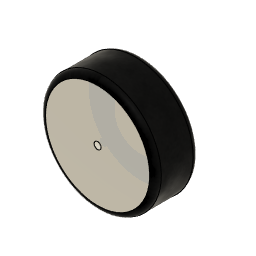
Robot v42 (Autodesk Fusion 360 archive; units mm, degrees)
design "Roues"
Autodesk Fusion 360 part; units mm, degrees
sketch "Esquisse1" plane through (0, 0, 0) normal (0, 1, 0) x (1, 0, 0)
  circle A0 centre (0, 0) radius 20
  circle A1 centre (0, 0) radius 3.1
  line L0 (-2.1, -2.2804) -> (-2.1, 2.2804)
  line L1 (2.1, -2.2804) -> (2.1, 2.2804)
  line L2 (0, 0) -> (0, -3.1) construction
  line L3 (0, 0) -> (0, 3.1) construction
  dimension "d1" = 40
  dimension "d4" = 6.2
  dimension "d5" = 4.2
  constraint coincident A0.centre A1.centre
  constraint concentric A0 A1
  constraint coincident A1 L0.start
  constraint coincident A1 L0.end
  constraint vertical L0
  constraint coincident A1 L1.start
  constraint coincident A1 L1.end
  constraint parallel L0 L1
  constraint coincident A1 L2.end
  constraint parallel L1 L2
  constraint coincident A1 L3.end
  constraint parallel L2 L3
  constraint symmetric L0 L1 L2
  measures "d1" diameter of A0
  measures "d4" diameter of A1
  measures "d5" distance of L0 L1
extrude "Extrusion1" add sketch "Esquisse1" along normal blind 7 contours A0 | A1 L1 | A1 L0
sketch "Esquisse2" plane through (0, 0, 0) normal (0, -1, 0) x (1, 0, 0)
  arc A0 (2.1, 2.2804) -> (-2.1, 2.2804) centre (0, 0) ccw
  line L0 (2.1, 2.2804) -> (2.1, -2.2804)
  arc A1 (-2.1, -2.2804) -> (2.1, -2.2804) centre (0, 0) ccw
  line L1 (-2.1, -2.2804) -> (-2.1, 2.2804)
  circle A2 centre (0, 0) radius 20
  constraint coincident A0.centre A1.centre
extrude "Extrusion2" add sketch "Esquisse2" against normal blind 4 contours A0 L0 A1 L1
hole "Perçage1" at (0, 0, 0) direction (0, 1, 0) diameter 2.4 depth 23 tip angle 118
sketch "Esquisse3" plane through (0, 7, 0) normal (0, 1, 0) x (-1, 0, 0)
  arc A0 (2.1, 2.2804) -> (-2.1, 2.2804) centre (0, 0) ccw
  line L0 (2.1, 2.2804) -> (2.1, -2.2804)
  arc A1 (-2.1, -2.2804) -> (2.1, -2.2804) centre (0, 0) ccw
  line L1 (-2.1, -2.2804) -> (-2.1, 2.2804)
  circle A2 centre (0, 0) radius 20
  arc A3 (2.1, 2.2804) -> (-2.1, 2.2804) centre (0, 0) ccw
  line L2 (-2.1, 2.2804) -> (-2.1, -2.2804)
  arc A4 (-2.1, -2.2804) -> (2.1, -2.2804) centre (0, 0) ccw
  line L3 (2.1, -2.2804) -> (2.1, 2.2804)
  arc A5 (-3.1, -2.6833) -> (3.1, -2.6833) centre (0, 0) ccw
  line L4 (3.1, 2.6833) -> (3.1, -2.6833)
  arc A6 (3.1, 2.6833) -> (-3.1, 2.6833) centre (0, 0) ccw
  line L5 (-3.1, -2.6833) -> (-3.1, 2.6833)
  circle A7 centre (0, 0) radius 1.2
  dimension "d11" = -1
extrude "Extrusion3" add sketch "Esquisse3" along normal blind 6 contours A5 L4 A6 L5
fillet "Congé1" radius 2 4 edges at (3.1, 10, 2.6833) (3.1, 10, -2.6833) (-3.1, 10, 2.6833) (-3.1, 10, -2.6833)
fillet "Congé2" radius 6 8 edges at (3.1, 7, 0) (2.8457, 7, 2.7648) (0, 7, 4.1) (-2.8457, 7, 2.7648) (-3.1, 7, 0) (-2.8457, 7, -2.7648) (0, 7, -4.1) (2.8457, 7, -2.7648)
sketch "Esquisse4" plane through (0, 7, 0) normal (0, 1, 0) x (-1, 0, 0)
  circle A0 centre (0, 0) radius 20
  line L0 (-9.1, -1.7889) -> (-9.1, 1.7889)
  arc A1 (-5.2905, 8.6035) -> (-9.1, 1.7889) centre (-1.1, 1.7889) ccw
  arc A2 (5.2905, 8.6035) -> (-5.2905, 8.6035) centre (0, 0) ccw
  arc A3 (9.1, 1.7889) -> (5.2905, 8.6035) centre (1.1, 1.7889) ccw
  line L1 (9.1, 1.7889) -> (9.1, -1.7889)
  arc A4 (5.2905, -8.6035) -> (9.1, -1.7889) centre (1.1, -1.7889) ccw
  arc A5 (-5.2905, -8.6035) -> (5.2905, -8.6035) centre (0, 0) ccw
  arc A6 (-9.1, -1.7889) -> (-5.2905, -8.6035) centre (-1.1, -1.7889) ccw
  circle A7 centre (0, 0) radius 20
  circle A8 centre (0, 0) radius 10.25
  line L2 (0, 0) -> (0, 20) construction
  line L3 (0, 10.25) -> (0, 20) construction
  circle A9 centre (0, 0) radius 18
  line L4 (2.5, 12) -> (2.5, 16)
  arc A10 (2.5, 16) -> (-2.5, 16) centre (0, 16) ccw
  line L5 (-2.5, 16) -> (-2.5, 12)
  arc A11 (-2.5, 12) -> (2.5, 12) centre (0, 12) ccw
  line L6 (0, 12) -> (0, 16) construction
  arc A12 (-1.5, 12) -> (1.5, 12) centre (0, 12) ccw
  line L7 (1.5, 12) -> (1.5, 16)
  arc A13 (1.5, 16) -> (-1.5, 16) centre (0, 16) ccw
  line L8 (-1.5, 16) -> (-1.5, 12)
  line L9 (-15.9894, 2.5666) -> (-12.1852, 1.3306)
  line L10 (-15.6804, 3.5177) -> (-11.8762, 2.2816)
  arc A14 (-14.7534, 6.3709) -> (-15.6804, 3.5177) centre (-15.2169, 4.9443) ccw
  arc A15 (-14.4444, 7.3219) -> (-15.9894, 2.5666) centre (-15.2169, 4.9443) ccw
  line L11 (-10.6401, 6.0858) -> (-14.4444, 7.3219)
  line L12 (-10.9492, 5.1348) -> (-14.7534, 6.3709)
  arc A16 (-11.8762, 2.2816) -> (-10.9492, 5.1348) centre (-11.4127, 3.7082) ccw
  arc A17 (-12.1852, 1.3306) -> (-10.6401, 6.0858) centre (-11.4127, 3.7082) ccw
  line L13 (-7.382, -14.4137) -> (-5.0309, -11.1777)
  line L14 (-8.191, -13.8259) -> (-5.8399, -10.5899)
  arc A18 (-10.6181, -12.0626) -> (-8.191, -13.8259) centre (-9.4046, -12.9443) ccw
  arc A19 (-11.4271, -11.4748) -> (-7.382, -14.4137) centre (-9.4046, -12.9443) ccw
  line L15 (-9.076, -8.2387) -> (-11.4271, -11.4748)
  line L16 (-8.2669, -8.8265) -> (-10.6181, -12.0626)
  arc A20 (-5.8399, -10.5899) -> (-8.2669, -8.8265) centre (-7.0534, -9.7082) ccw
  arc A21 (-5.0309, -11.1777) -> (-9.076, -8.2387) centre (-7.0534, -9.7082) ccw
  line L17 (11.4271, -11.4748) -> (9.076, -8.2387)
  line L18 (10.6181, -12.0626) -> (8.2669, -8.8265)
  arc A22 (8.191, -13.8259) -> (10.6181, -12.0626) centre (9.4046, -12.9443) ccw
  arc A23 (7.382, -14.4137) -> (11.4271, -11.4748) centre (9.4046, -12.9443) ccw
  line L19 (5.0309, -11.1777) -> (7.382, -14.4137)
  line L20 (5.8399, -10.5899) -> (8.191, -13.8259)
  arc A24 (8.2669, -8.8265) -> (5.8399, -10.5899) centre (7.0534, -9.7082) ccw
  arc A25 (9.076, -8.2387) -> (5.0309, -11.1777) centre (7.0534, -9.7082) ccw
  line L21 (14.4444, 7.3219) -> (10.6401, 6.0858)
  line L22 (14.7534, 6.3709) -> (10.9492, 5.1348)
  arc A26 (15.6804, 3.5177) -> (14.7534, 6.3709) centre (15.2169, 4.9443) ccw
  arc A27 (15.9894, 2.5666) -> (14.4444, 7.3219) centre (15.2169, 4.9443) ccw
  line L23 (12.1852, 1.3306) -> (15.9894, 2.5666)
  line L24 (11.8762, 2.2816) -> (15.6804, 3.5177)
  arc A28 (10.9492, 5.1348) -> (11.8762, 2.2816) centre (11.4127, 3.7082) ccw
  arc A29 (10.6401, 6.0858) -> (12.1852, 1.3306) centre (11.4127, 3.7082) ccw
  dimension "d18" = 20.5
  dimension "d19" = -2
  dimension "d20" = 16
  dimension "d21" = 12
  dimension "d22" = 5
  dimension "d23" = -1
  dimension "d25" = 360
  constraint concentric A7 A8
  constraint coincident A0.centre A2.centre
  constraint coincident A7 L2.end
  constraint vertical L2
  constraint coincident A8 L3.start
  constraint coincident L2 L3.start
  constraint tangent L4 A10
  constraint tangent A10 L5
  constraint parallel L4 L5
  constraint tangent L5 A11
  constraint tangent L4 A11
  constraint coincident L2 A10.centre
  constraint parallel L2 L6
  measures "d18" diameter of A8
  measures "d20" distance of A0.centre A10.centre
  measures "d21" distance of A0.centre A11.centre
  measures "d22" distance of L4 L5
extrude "Extrusion5" add 1 faces at (13.6578, 0, 1.0235) along direction (0, -1, 0) blind 3
extrude "Extrusion6" add 1 faces at (13.6578, -3, 1.0235) along direction (0, -1, 0) blind 5
extrude "Extrusion7" cut 1 faces at (-1.7989, 4, 0.0299) along direction (0, -1, 0) blind 10
fillet "Congé4" radius 2 2 edges at (-18.6465, -8, -7.2323) (-18.6465, 7, 7.2323)

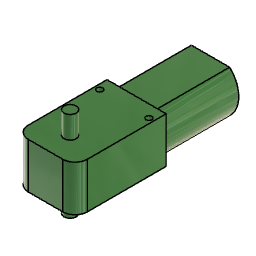
design "Moteur dc"
Autodesk Fusion 360 part; units mm, degrees
sketch "Esquisse1" plane through (0, 0, 0) normal (0, 1, 0) x (1, 0, 0)
  circle A0 centre (0, 0) radius 11.5
  line L0 (-7.746, 8.5) -> (7.746, 8.5)
  line L1 (-7.746, -8.5) -> (7.746, -8.5)
  line L2 (0, 0) -> (-11.5, 0) construction
  line L3 (0, 0) -> (11.5, 0) construction
  dimension "d1" = 23
  dimension "d2" = 17
  constraint coincident A0.centre L2.start
  constraint coincident A0 L0.start
  constraint coincident A0 L0.end
  constraint horizontal L0
  constraint coincident A0 L1.start
  constraint coincident A0 L1.end
  constraint parallel L0 L1
  constraint coincident A0 L2.end
  constraint horizontal L2
  constraint coincident A0 L3.end
  constraint parallel L2 L3
  constraint symmetric L0 L1 L3
  measures "d1" diameter of A0
  measures "d2" distance of L0 L1
extrude "Extrusion1" add sketch "Esquisse1" along normal blind 30 contours A0 L0 L1
sketch "Esquisse2" plane through (0, 0, 0) normal (0, -1, 0) x (1, 0, 0)
  arc A0 (-7.746, 8.5) -> (-7.746, -8.5) centre (0, 0) ccw
  line L0 (-7.746, -8.5) -> (7.746, -8.5)
  arc A1 (7.746, -8.5) -> (7.746, 8.5) centre (0, 0) ccw
  line L1 (7.746, 8.5) -> (-7.746, 8.5)
  line L2 (12, 9.25) -> (-12, 9.25)
  line L3 (-12, 9.25) -> (-12, -9.25)
  line L4 (-12, -9.25) -> (12, -9.25)
  line L5 (12, -9.25) -> (12, 9.25)
  line L6 (12, 9.25) -> (-12, -9.25) construction
  line L7 (-12, 9.25) -> (12, -9.25) construction
  dimension "d5" = 18.5
  dimension "d6" = 24
  constraint horizontal L2
  constraint perpendicular L2 L3
  constraint parallel L2 L4
  constraint parallel L3 L5
  constraint coincident L6 A0.centre
  constraint coincident L7 A0.centre
  constraint coincident A0.centre A1.centre
  measures "d5" distance of L2.end L3.end
  measures "d6" distance of L2.start L2.end
extrude "Extrusion2" add sketch "Esquisse2" along normal blind 37 contours A0 L0 A1 L1 | L2 L3 L4 L5
fillet "Congé1" radius 5 2 edges at (12, -37, 0) (-12, -37, 0)
sketch "Esquisse3" plane through (0, 0, 9.25) normal (0, 0, 1) x (-1, 0, 0)
  arc A0 (12, 32) -> (7, 37) centre (7, 32) ccw
  line L0 (7, 37) -> (-7, 37)
  arc A1 (-7, 37) -> (-12, 32) centre (-7, 32) ccw
  line L1 (-12, 32) -> (-12, 0)
  line L2 (-12, 0) -> (12, 0)
  line L3 (12, 0) -> (12, 32)
  line L4 (12, 27) -> (-12, 27) construction
  circle A2 centre (0, 27) radius 2.5
  dimension "d11" = 10
  dimension "d12" = 5
  constraint coincident L3 L4.start
  constraint coincident L1 L4.end
  constraint perpendicular L1 L4
  constraint midpoint L4 A2.centre
  measures "d11" distance of L0 L4
  measures "d12" diameter of A2
extrude "Extrusion3" add sketch "Esquisse3" along normal blind 9 contours A2
ref_plane "Plan de construction1" through (0, -18.5, 0) normal (0, 0, 1) x (-1, 0, 0)
mirror "Symétrie miroir1" about plane through (0, -18.5, 0) normal (0, 0, 1) of "Extrusion3"
sketch "Esquisse4" plane through (0, 0, 9.25) normal (0, 0, 1) x (-1, 0, 0)
  circle A0 centre (0, 27) radius 2.5
  arc A1 (12, 32) -> (7, 37) centre (7, 32) ccw
  line L0 (7, 37) -> (-7, 37)
  arc A2 (-7, 37) -> (-12, 32) centre (-7, 32) ccw
  line L1 (-12, 32) -> (-12, 0)
  line L2 (-12, 0) -> (12, 0)
  line L3 (12, 0) -> (12, 32)
  line L4 (12, 5) -> (-12, 5) construction
  line L5 (-12, 0) -> (12, 0)
  line L6 (0, 0) -> (0, 37) construction
  point P0 (10, 5)
  point P1 (-10, 5)
  dimension "d17" = 5
  dimension "d18" = 2
  constraint coincident L3 L4.start
  constraint coincident L1 L4.end
  constraint perpendicular L1 L4
  constraint coincident L6.start origin
  constraint midpoint L0 L6.end
  constraint coincident L4 P0
  constraint symmetric L6 P0 P1
  measures "d17" distance of L4 L5
  measures "d18" distance of L3 P0
hole "Perçage1" at (-10, -5, 9.25) at (10, -5, 9.25) direction (0, 0, -1) diameter 2.4 depth 42 tip angle 118
sketch "Esquisse5" plane through (0, 0, 9.25) normal (0, 0, 1) x (-1, 0, 0)
  circle A0 centre (10, 5) radius 1.2
  circle A1 centre (-10, 5) radius 1.2
  circle A2 centre (0, 27) radius 2.5
  arc A3 (12, 32) -> (7, 37) centre (7, 32) ccw
  line L0 (7, 37) -> (-7, 37)
  arc A4 (-7, 37) -> (-12, 32) centre (-7, 32) ccw
  line L1 (-12, 32) -> (-12, 0)
  line L2 (-12, 0) -> (12, 0)
  line L3 (12, 0) -> (12, 32)
  line L4 (7.746, 0) -> (-7.746, 0)
  line L5 (-7.746, 0) -> (-7.746, -30)
  line L6 (-7.746, -30) -> (7.746, -30)
  line L7 (7.746, -30) -> (7.746, 0)
  line L8 (-7, 37) -> (7, 37)
  line L9 (0, -30) -> (0, 37)
  circle A5 centre (0, 27) radius 2.5
  point P0 (0, 3.5)
  dimension "d22" = 10
  dimension "d23" = 1.5
  dimension "d24" = 1.5
  dimension "d25" = 12
  dimension "d26" = 23.5
  dimension "d26" = 23.5
  constraint midpoint L6 L9.start
  constraint midpoint L8 L9.end
  constraint midpoint L9 P0
  measures "d22" horizontal distance of A0.centre P0
  measures "d23" vertical distance of A0.centre P0
  measures "d24" vertical distance of A1.centre P0
  measures "d25" distance of L3 P0
  measures "d26" distance of A2.centre P0

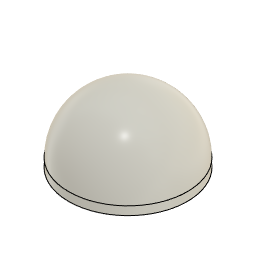
design "Bille"
Autodesk Fusion 360 part; units mm, degrees
sketch "Esquisse1" plane through (0, 0, 0) normal (0, 0, 1) x (1, 0, 0)
  circle A0 centre (0, 0) radius 7
  line L0 (0, 0) -> (0, 7)
  line L1 (0, 0) -> (0, -7)
  dimension "d1" = 14
  constraint coincident A0.centre L0.start
  constraint coincident A0 L0.end
  constraint vertical L0
  constraint coincident A0 L1.end
  constraint parallel L0 L1
  measures "d1" diameter of A0
revolve "Révolution1" add sketch "Esquisse1" angle 180 about axis through (0, 0, 0) along (0, 1, 0) contours A0 L0 L1 picked at (-0.3478, -4.6406)
extrude "Extrusion1" add 2 faces at (-0.3478, -4.6406, 0) (0.3478, -4.6406, 0) along direction (0, 0, -1) blind 1
